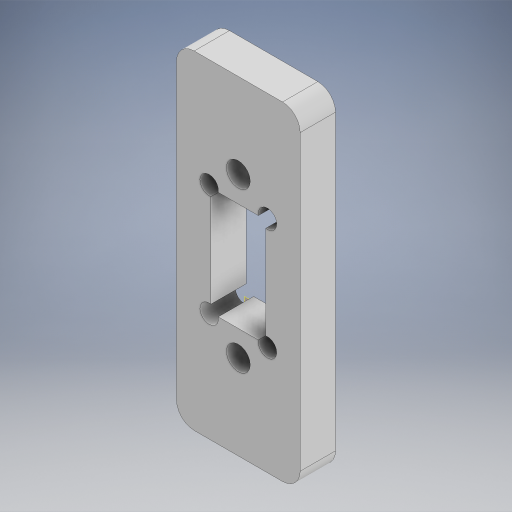
# Autodesk Inventor part: body front connection_zig3
Saved by Autodesk Inventor 2024 (Build 280153000, 153)
## iProperties
Created: 2024-09-11
Part Number: body front connection_zig3
Material: 일반
Document SubType Name: Modeling
Designer: ASUS
Density: 1 g/cm^3
Appearance: 기본값
Author: ASUS
Autodesk Inventor part; units mm, degrees
ref_plane "YZ Plane" through (0, 0, 0) normal (1, 0, 0) x (0, 1, 0)
ref_plane "XZ Plane" through (0, 0, 0) normal (0, 1, 0) x (-1, 0, 0)
ref_plane "XY Plane" through (0, 0, 0) normal (0, 0, 1) x (1, 0, 0)
ref_plane "작업 평면1" through (0, -20.6, 0) normal (0, 0, 1) x (1, 0, 0)
sketch "스케치1" plane through (0, -20.6, 0) normal (0, 0, 1) x (1, 0, 0)
  line L0 (0, 13) -> (6, 13) projected
  line L1 (6, 20.6) -> (6, 13) projected
  line L2 (0, 20.6) -> (6, 20.6) projected
  line L3 (0, 20.6) -> (0, 13) projected
  circle A0 centre (3, 15) radius 1.35 projected
  line L4 (0, 12) -> (0, 0) projected
  line L5 (0, 0) -> (6, 0) projected
  line L6 (6, 12) -> (6, 0) projected
  line L7 (0, 12) -> (6, 12) projected
  line L8 (6, -1) -> (0, -1) projected
  line L9 (0, -1) -> (0, -8.6) projected
  line L10 (0, -8.6) -> (6, -8.6) projected
  line L11 (6, -1) -> (6, -8.6) projected
  circle A1 centre (3, -3) radius 1.35 projected
  line L12 (6.3, -0.3) -> (-0.3, -0.3)
  line L13 (-0.3, -0.3) -> (-0.3, 12.3)
  line L14 (-0.3, 12.3) -> (6.3, 12.3)
  line L15 (6.3, 12.3) -> (6.3, -0.3)
  circle A2 centre (6.3, 12.3) radius 0.75
  circle A3 centre (-0.3, 12.3) radius 0.75
  circle A4 centre (6.3, -0.3) radius 0.75
  circle A5 centre (-0.3, -0.3) radius 0.75
  line L16 (6, 20.6) -> (0, 20.6)
  line L17 (0, 20.6) -> (0, -8.6)
  line L18 (0, -8.6) -> (6, -8.6)
  line L19 (6, -8.6) -> (6, 20.6)
  line L20 (10, 24.6) -> (-4, 24.6)
  line L21 (-4, 24.6) -> (-4, -12.6)
  line L22 (-4, -12.6) -> (10, -12.6)
  line L23 (10, -12.6) -> (10, 24.6)
  point P0 (0.45, 12.3)
  point P1 (5.55, 12.3)
  point P2 (6.3, 11.55)
  point P3 (6.3, 0.45)
  point P4 (5.55, -0.3)
  point P5 (0.45, -0.3)
  point P6 (-0.3, 0.45)
  point P7 (-0.3, 11.55)
  dimension "d0" = 0.3
  dimension "d1" = 1.5
  dimension "d2" = 1.5
  dimension "d3" = 1.5
  dimension "d4" = 1.5
  dimension "d5" = 4
  constraints: 24 end point, 4 centre point, 4 coincident, 4 parallel, 2 perpendicular, 1 horizontal, 6 other
  measures "d0" distance between parallel lines of L6 L15
  measures "d1" diameter of A2
  measures "d2" diameter of A3
  measures "d3" diameter of A4
  measures "d4" diameter of A5
  measures "d5" distance between parallel lines of L19 L23
extrude "돌출1" add sketch "스케치1" along normal blind 4 contours L3 L2 L1 L0 | L0 L19 A2 L14 A3 L17 | A5 L12 A4 L19 L8 L17 | L8 L11 L10 L9 | L23 L22 L21 L20
fillet "모깎기1" radius 2 4 edges at (-4, 4, 2) (10, 4, 2) (10, -33.2, 2) (-4, -33.2, 2)
sketch "스케치2" plane through (0, -20.6, 4) normal (0, 0, 1) x (1, 0, 0)
  arc A0 (-4, -10.6) -> (-2, -12.6) centre (-2, -10.6) ccw projected
  line L0 (-2, -12.6) -> (8, -12.6) projected
  arc A1 (8, -12.6) -> (10, -10.6) centre (8, -10.6) ccw projected
  line L1 (10, -10.6) -> (10, 22.6) projected
  arc A2 (10, 22.6) -> (8, 24.6) centre (8, 22.6) ccw projected
  line L2 (8, 24.6) -> (-2, 24.6) projected
  arc A3 (-2, 24.6) -> (-4, 22.6) centre (-2, 22.6) ccw projected
  line L3 (-4, 22.6) -> (-4, -10.6) projected
  circle A4 centre (3, 15) radius 1.35 projected
  arc A5 (0.45, 12.3) -> (-0.3, 11.55) centre (-0.3, 12.3) ccw projected
  line L4 (0.45, 12.3) -> (5.55, 12.3) projected
  arc A6 (6.3, 11.55) -> (5.55, 12.3) centre (6.3, 12.3) ccw projected
  line L5 (6.3, 11.55) -> (6.3, 0.45) projected
  arc A7 (5.55, -0.3) -> (6.3, 0.45) centre (6.3, -0.3) ccw projected
  line L6 (5.55, -0.3) -> (0.45, -0.3) projected
  arc A8 (-0.3, 0.45) -> (0.45, -0.3) centre (-0.3, -0.3) ccw projected
  line L7 (-0.3, 0.45) -> (-0.3, 11.55) projected
  circle A9 centre (3, -3) radius 1.35 projected
  line L8 (6.1, 0.2123) -> (6.1, 11.7877)
  arc A10 (6.1, 11.7877) -> (5.7877, 12.1) centre (6.3, 12.3) ccw
  line L9 (5.7877, 12.1) -> (0.2123, 12.1)
  arc A11 (0.2123, 12.1) -> (-0.1, 11.7877) centre (-0.3, 12.3) ccw
  line L10 (-0.1, 11.7877) -> (-0.1, 0.2123)
  arc A12 (-0.1, 0.2123) -> (0.2123, -0.1) centre (-0.3, -0.3) ccw
  line L11 (0.2123, -0.1) -> (5.7877, -0.1)
  arc A13 (5.7877, -0.1) -> (6.1, 0.2123) centre (6.3, -0.3) ccw
  point P0 (0, 20.6)
  dimension "d9" = 0.2
  constraints: 8 end point, 8 point on circle, 4 centre point, 7 other
  measures "d9" distance between parallel lines of L5 L8
extrude "돌출2" add sketch "스케치2" against normal up to surface (4 mm away) contours L4 A6 L5 A7 L6 A8 L7 A5
sketch "스케치3" plane through (0, -20.6, 4) normal (0, 0, 1) x (1, 0, 0)
  arc A0 (5.7877, -0.1) -> (6.1, 0.2123) centre (6.3, -0.3) ccw projected
  line L0 (5.7877, -0.1) -> (0.2123, -0.1) projected
  arc A1 (-0.1, 0.2123) -> (0.2123, -0.1) centre (-0.3, -0.3) ccw projected
  line L1 (-0.1, 0.2123) -> (-0.1, 11.7877) projected
  arc A2 (0.2123, 12.1) -> (-0.1, 11.7877) centre (-0.3, 12.3) ccw projected
  line L2 (0.2123, 12.1) -> (5.7877, 12.1) projected
  arc A3 (6.1, 11.7877) -> (5.7877, 12.1) centre (6.3, 12.3) ccw projected
  line L3 (6.1, 11.7877) -> (6.1, 0.2123) projected
  arc A4 (-4, -10.6) -> (-2, -12.6) centre (-2, -10.6) ccw projected
  line L4 (-2, -12.6) -> (8, -12.6) projected
  arc A5 (8, -12.6) -> (10, -10.6) centre (8, -10.6) ccw projected
  line L5 (10, -10.6) -> (10, 22.6) projected
  arc A6 (10, 22.6) -> (8, 24.6) centre (8, 22.6) ccw projected
  line L6 (8, 24.6) -> (-2, 24.6) projected
  arc A7 (-2, 24.6) -> (-4, 22.6) centre (-2, 22.6) ccw projected
  line L7 (-4, 22.6) -> (-4, -10.6) projected
  circle A8 centre (3, 15) radius 1.35 projected
  circle A9 centre (3, -3) radius 1.35 projected
  point P0 (0, 20.6)
hole "구멍1" at (6.3, -20.9, 4) at (6.3, -8.3, 4) at (-0.3, -8.3, 4) at (-0.3, -20.9, 4) direction (0, 0, -1) diameter 2.1 end through all
